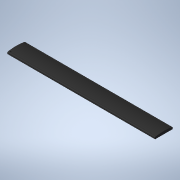
# Autodesk Inventor part: ETH2-17-350_3
Saved by Autodesk Inventor 2021 (Build 250183000, 183)
## iProperties
Created: 2025-05-01
Part Number: ETH2-17-350_3
Material: Generic
Catalog Web Link: www.cadenas.de
Description: ETH2_17_3-ETH2
Vendor: TOYO
Document SubType Name: Modeling
Designer: psAdmin
Manufacturer: TOYO
Mass: 436.332 g
Surface Area: 953.902 cm^2
Volume: 436.332 cm^3
Density: 1 g/cm^3
Appearance: PSOLRGB-175-175-175
Category: PARTsolutions
Company: TOYO
Title: ETH2-17-350
Author: Cadenas PARTsolutions
Comments: ETH2
PSOL_IDENT_0: {$CADENAS_DATA/23d-libs/toyo/eth2_series/eth2_17/parts/eth2_17_body3.prj},179 {VTYP=3D},{NB=ETH2-17-
PSOL_IDENT_1: 350_3},{LINA=ETH2-17-350},{NN=ETH2_17_3},{DATE=02.07.2024 05:59:00},{GEOMDATE=05.06.2024 08:29:00},{
PSOL_IDENT_2: VERSION=},{LINEID=10},{WBVAR=STROKE},{WBNUMERIC=STROKE}  {NB=ETH2-17-350_3},{LINA=ETH2-17-350},{KT=D
PSOL_IDENT_3: UMMY},{CNSORDERNO=ETH2-17-350},{MODEL=ETH2-17},{STROKE=350}
NB: ETH2-17-350_3
NN: ETH2_17_3
NT: ETH2
NBSYN: $CNSORDERNO._3
LINA: ETH2-17-350
CATALOG: TOYO
MODEL: ETH2-17
STROKE: 350
SUPPLIER: TOYO
ARTICLENO: ETH2-17-350_3
BOMINFO: ETH2-17-350
CREATOR: CADENAS GmbH
Autodesk Inventor part; units mm, degrees
sketch "__2" plane through (0, 0, 0) normal (1, 0, 0) x (0, 1, 0)
  arc A0 (0.5, 35.5) -> (0, 35) centre (0.5, 35) ccw
  line L0 (0, 35) -> (0, -35)
  arc A1 (0, -35) -> (0.5, -35.5) centre (0.5, -35) ccw
  line L1 (0.5, -35.5) -> (6.3099, -35.5)
  arc A2 (6.3099, -35.5) -> (8.274, -33.877) centre (6.3099, -33.5) ccw
  arc A3 (8.274, -33.877) -> (8.7, -31.581) centre (-167.9972, 0.0159) ccw
  line L2 (8.7, -31.581) -> (8.7, -29.75)
  line L3 (8.7, -29.75) -> (9.051, -29.547)
  arc A4 (9.051, -29.547) -> (9.051, 29.547) centre (-168.0005, 0) ccw
  line L4 (9.051, 29.547) -> (8.7, 29.75)
  line L5 (8.7, 29.75) -> (8.7, 31.581)
  arc A5 (8.7, 31.581) -> (8.274, 33.877) centre (-167.9972, -0.0159) ccw
  arc A6 (8.274, 33.877) -> (6.3099, 35.5) centre (6.3099, 33.5) ccw
  line L6 (6.3099, 35.5) -> (0.5, 35.5)
  constraints: 14 end point, 14 point on circle, 7 centre point
extrude "Extrusion1" add sketch "__2" along normal blind 597
sketch "__1" plane through (0, 7.18, 0) normal (0, 1, 0) x (1, 0, 0)
  circle A0 centre (8, 30.29) radius 3.25
  constraints: 1 centre point
extrude "Extrusion2" cut sketch "__1" along normal blind 3.52
pattern_linear "Rectangular Pattern1" count 2 spacing 631 along (1, 0, 0) count 2 spacing 60.58 along (0, 0, 1) of "Extrusion2"
ref_plane "BODYS_XY" through (0, 0, 0) normal (1, 0, 0) x (0, 0, -1)
ref_plane "BODYS_YZ" through (0, 0, 0) normal (0, 0, -1) x (0, 1, 0)
ref_plane "BODYS_ZX" through (0, 0, 0) normal (0, 1, 0) x (1, 0, 0)
body "Solid1"
